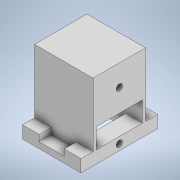
# Autodesk Inventor part: support servo
Saved by Autodesk Inventor 2022 (Build 260153000, 153)
## iProperties
Created: 2022-04-29
Part Number: support servo
Material: Generic
Document SubType Name: Modeling
Designer: Oana
Density: 1 g/cm^3
Appearance: Default
Author: Oana
Autodesk Inventor part; units mm, degrees
ref_plane "YZ Plane" through (0, 0, 0) normal (1, 0, 0) x (0, 1, 0)
ref_plane "XZ Plane" through (0, 0, 0) normal (0, 1, 0) x (-1, 0, 0)
ref_plane "XY Plane" through (0, 0, 0) normal (0, 0, 1) x (1, 0, 0)
sketch "Sketch1" plane through (0, 0, 0) normal (0, 1, 0) x (-1, 0, 0)
  line L0 (6.2884, 19.9233) -> (-5.9116, 19.9233)
  line L1 (-5.9116, 19.9233) -> (-5.9116, 12.6233)
  line L2 (-5.9116, 12.6233) -> (6.2884, 12.6233)
  line L3 (6.2884, 12.6233) -> (6.2884, 19.9233)
  point P0 (0, 0)
  dimension "d0" = 7.3
  dimension "d1" = 12.2
  constraints: 8 end point, 2 parallel, 1 horizontal, 1 perpendicular
  measures "d0" distance of L2.end L0.start
  measures "d1" distance of L0.start L0.end
extrude "Extrusion1" add sketch "Sketch1" along normal blind 3
sketch "Sketch2" plane through (0, 3, 0) normal (0, 1, 0) x (1, 0, 0)
  line L0 (5.9116, -19.9233) -> (5.9116, -12.6233) projected
  line L1 (5.9116, -12.6233) -> (-6.2884, -12.6233) projected
  line L2 (-6.2884, -12.6233) -> (-6.2884, -19.9233) projected
  line L3 (-6.2884, -19.9233) -> (5.9116, -19.9233) projected
  line L4 (5.9116, -12.6233) -> (-6.2884, -12.6233)
  line L5 (-6.2884, -12.6233) -> (-6.2884, -14.1233)
  line L6 (-6.2884, -14.1233) -> (5.9116, -14.1233)
  line L7 (5.9116, -14.1233) -> (5.9116, -12.6233)
  point P0 (0, 0)
  point P1 (5.9116, -14.1233)
  dimension "d4" = 1.5
  constraints: 8 end point, 2 parallel, 1 horizontal, 1 perpendicular, 1 point on line
  measures "d4" distance between parallel lines of L1 L6
extrude "Extrusion2" add sketch "Sketch2" along normal blind 15.7 contours L6 L2 L1 L0
sketch "Sketch3" plane through (5.9116, 0, 12.6233) normal (0, 0, -1) x (-1, 0, 0)
  line L0 (0, 0) -> (12.2, 0) projected
  line L1 (12.2, 0) -> (12.2, 18.7) projected
  line L2 (0, 18.7) -> (12.2, 18.7) projected
  line L3 (0, 0) -> (0, 18.7) projected
  line L4 (0, 18.7) -> (12.2, 18.7)
  line L5 (12.2, 18.7) -> (12.2, 15.7)
  line L6 (12.2, 15.7) -> (0, 15.7)
  line L7 (0, 15.7) -> (0, 18.7)
  point P0 (5.9116, 0)
  point P1 (0, 15.7)
  dimension "d7" = 3
  constraints: 8 end point, 2 parallel, 1 horizontal, 1 perpendicular, 1 point on line
  measures "d7" distance between parallel lines of L2 L6
extrude "Extrusion3" add sketch "Sketch3" along normal blind 23.8 contours L3 L2 L1 L6
sketch "Sketch4" plane through (-6.2884, 15.7, 12.6233) normal (0, -1, 0) x (1, 0, 0)
  line L0 (0, 0) -> (12.2, 0) projected
  line L1 (0, 0) -> (0, -23.8) projected
  line L2 (12.2, -23.8) -> (0, -23.8) projected
  line L3 (12.2, 0) -> (12.2, -23.8) projected
  line L4 (12.2, -23.8) -> (0, -23.8)
  line L5 (0, -23.8) -> (0, -22.3)
  line L6 (0, -22.3) -> (12.2, -22.3)
  line L7 (12.2, -22.3) -> (12.2, -23.8)
  point P0 (6.2884, -12.6233)
  dimension "d10" = 1.5
  constraints: 8 end point, 2 parallel, 1 horizontal, 1 perpendicular, 1 point on line
  measures "d10" distance between parallel lines of L2 L6
extrude "Extrusion4" add sketch "Sketch4" along normal up to surface (15.7 mm away) contours L6 L3 L2 L1
sketch "Sketch5" plane through (5.9116, 0, -11.1767) normal (0, 0, -1) x (-1, 0, 0)
  line L0 (12.2, 18.7) -> (12.2, 0) projected
  line L1 (12.2, 18.7) -> (0, 18.7) projected
  line L2 (0, 18.7) -> (0, 0) projected
  line L3 (12.2, 0) -> (0, 0) projected
  line L4 (12.2, 0) -> (0, 0)
  line L5 (0, 0) -> (0, 3)
  line L6 (0, 3) -> (12.2, 3)
  line L7 (12.2, 3) -> (12.2, 0)
  point P0 (5.9116, 0)
  dimension "d13" = 3
  constraints: 8 end point, 2 parallel, 1 horizontal, 1 perpendicular, 1 point on line
  measures "d13" distance between parallel lines of L3 L6
extrude "Extrusion5" add sketch "Sketch5" along normal blind 5.8 contours L0 L3 L2 L6
sketch "Sketch6" plane through (0, 0, 0) normal (0, -1, 0) x (1, 0, 0)
  arc A0 (-0.7384, -2.4741) -> (0.3616, -2.4741) centre (-0.1884, -3.4267) ccw construction
  circle A1 centre (-0.1884, -3.4267) radius 1.1 construction
  arc A2 (0.3616, -32.1794) -> (-0.7384, -32.1794) centre (-0.1884, -31.2267) ccw projected
  circle A3 centre (-0.1884, -31.2267) radius 1.5
  circle A4 centre (-0.1884, -3.4267) radius 1.5
  point P0 (0, 0)
  dimension "d16" = 3
  dimension "d17" = 3
  constraints: 3 centre point, 3 coincident, 1 concentric, 1 other
  measures "d16" diameter of A3
  measures "d17" diameter of A4
extrude "Extrusion6" cut sketch "Sketch6" against normal up to surface (3 mm away)
sketch "Sketch8" plane through (5.9116, 0, 19.9233) normal (1, 0, 0) x (0, 0, -1)
  line L0 (0, 0) -> (7.3, 0) projected
  line L1 (7.3, 0) -> (7.3, 15.7) projected
  line L2 (7.3, 15.7) -> (29.6, 15.7) projected
  line L3 (29.6, 15.7) -> (29.6, 0) projected
  line L4 (36.9, 0) -> (29.6, 0) projected
  line L5 (36.9, 3) -> (36.9, 0) projected
  line L6 (31.1, 3) -> (36.9, 3) projected
  line L7 (31.1, 18.7) -> (31.1, 3) projected
  line L8 (5.8, 18.7) -> (31.1, 18.7) projected
  line L9 (5.8, 3) -> (5.8, 18.7) projected
  line L10 (0, 3) -> (5.8, 3) projected
  line L11 (0, 0) -> (0, 3) projected
  line L12 (0, 0) -> (36.9, 0)
  line L13 (36.9, 0) -> (36.9, 6)
  line L14 (36.9, 6) -> (0, 6)
  line L15 (0, 6) -> (0, 0)
  point P0 (19.9233, 0)
  dimension "d22" = 6
  constraints: 8 end point, 2 parallel, 1 horizontal, 1 perpendicular
  measures "d22" distance of L14.end L0.start
extrude "Extrusion8" add sketch "Sketch8" along normal blind 8 contours L11 L10 L9 L14 L1 L0 | L1 L14 L3 L12 | L15 L14 L9 L10 | L3 L14 L7 L6 L5 L4 | L14 L13 L6 L7
sketch "Sketch9" plane through (-6.2884, 0, 12.6233) normal (-1, 0, 0) x (0, 0, 1)
  line L0 (-29.6, 6) -> (7.3, 6)
  line L1 (7.3, 6) -> (7.3, 0)
  line L2 (7.3, 0) -> (-29.6, 0)
  line L3 (-29.6, 0) -> (-29.6, 6)
  point P0 (-12.6233, 0)
  point P1 (7.3, 6)
  point P2 (-29.6, 0)
  constraints: 8 end point, 2 parallel, 1 horizontal, 1 perpendicular
extrude "Extrusion9" add sketch "Sketch9" along normal blind 8
sketch "Sketch10" plane through (13.9116, 0, 19.9233) normal (1, 0, 0) x (0, 0, -1)
  line L0 (0, 6) -> (0, 0) projected
  line L1 (0, 0) -> (36.9, 0) projected
  line L2 (36.9, 0) -> (36.9, 6) projected
  line L3 (36.9, 6) -> (0, 6) projected
  line L4 (0, 6) -> (36.9, 0) construction
  line L5 (36.9, 6) -> (0, 0) construction
  circle A0 centre (18.45, 3) radius 1.5
  point P0 (19.9233, 0)
  dimension "d27" = 3
  constraints: 4 end point, 1 centre point, 1 midpoint
  measures "d27" diameter of A0
extrude "Extrusion10" cut sketch "Sketch10" against normal blind 8 contours A0
sketch "Sketch11" plane through (0, 18.7, 0) normal (0, 1, 0) x (1, 0, 0)
  line L0 (5.9116, -14.1233) -> (5.9116, 11.1767) projected
  line L1 (-6.2884, 11.1767) -> (5.9116, 11.1767) projected
  line L2 (-6.2884, -14.1233) -> (-6.2884, 11.1767) projected
  line L3 (-6.2884, -14.1233) -> (5.9116, -14.1233) projected
  line L4 (5.9116, -14.1233) -> (0, -14.1233)
  line L5 (0, -14.1233) -> (0, 11.1767)
  line L6 (0, 11.1767) -> (5.9116, 11.1767)
  line L7 (5.9116, 11.1767) -> (5.9116, -14.1233)
  point P0 (0, 0)
  constraints: 8 end point, 2 parallel, 1 horizontal, 1 perpendicular, 1 point on line
extrude "Extrusion11" add sketch "Sketch11" along normal blind 10 contours L3 L5 L1 L0
sketch "Sketch12" plane through (5.9116, 15.7, 12.6233) normal (1, 0, 0) x (0, 0, -1)
  line L0 (22.3, -9.7) -> (23.8, -9.7) projected
  line L1 (23.8, -9.7) -> (23.8, 13) projected
  line L2 (-1.5, 13) -> (23.8, 13) projected
  line L3 (-1.5, -9.7) -> (-1.5, 13) projected
  line L4 (-1.5, -9.7) -> (0, -9.7) projected
  line L5 (0, -9.7) -> (0, 0) projected
  line L6 (0, 0) -> (22.3, 0) projected
  line L7 (22.3, 0) -> (22.3, -9.7) projected
  line L8 (-1.5, 13) -> (23.8, 13)
  line L9 (23.8, 13) -> (23.8, 5)
  line L10 (23.8, 5) -> (-1.5, 5)
  line L11 (-1.5, 5) -> (-1.5, 13)
  point P0 (12.6233, -15.7)
  point P1 (-1.5, 5)
  dimension "d32" = 8
  constraints: 8 end point, 2 parallel, 1 horizontal, 1 perpendicular, 1 point on line
  measures "d32" distance between parallel lines of L2 L10
extrude "Extrusion12" add sketch "Sketch12" along normal up to surface (8 mm away) contours L10 L3 L2 L1
sketch "Sketch14" plane through (0, 28.7, 0) normal (0, 1, 0) x (1, 0, 0)
  line L0 (5.9116, 11.1767) -> (5.9116, -14.1233) projected
  line L1 (0, -14.1233) -> (13.9116, -14.1233) projected
  line L2 (13.9116, -14.1233) -> (13.9116, 11.1767) projected
  line L3 (0, 11.1767) -> (13.9116, 11.1767) projected
  line L4 (0, 11.1767) -> (0, -14.1233) projected
  line L5 (0, 11.1767) -> (13.9116, 11.1767)
  line L6 (13.9116, 11.1767) -> (13.9116, -14.1233)
  line L7 (13.9116, -14.1233) -> (0, -14.1233)
  line L8 (0, -14.1233) -> (0, 11.1767)
  point P0 (0, 0)
  constraints: 8 end point, 2 parallel, 1 horizontal, 1 perpendicular
extrude "Extrusion14" add sketch "Sketch14" along normal blind 8
sketch "Sketch16" plane through (5.9116, 15.7, 12.6233) normal (1, 0, 0) x (0, 0, -1)
  line L0 (23.8, 5) -> (-1.5, 5) projected
  line L1 (-1.5, -9.7) -> (-1.5, 5) projected
  line L2 (-1.5, -9.7) -> (0, -9.7) projected
  line L3 (0, -9.7) -> (0, 0) projected
  line L4 (0, 0) -> (22.3, 0) projected
  line L5 (22.3, 0) -> (22.3, -9.7) projected
  line L6 (22.3, -9.7) -> (23.8, -9.7) projected
  line L7 (23.8, -9.7) -> (23.8, 5) projected
  point P0 (12.6233, -15.7)
extrude "Extrusion16" add sketch "Sketch16" along normal blind 8
sketch "Sketch17" plane through (13.9116, 0, 19.9233) normal (1, 0, 0) x (0, 0, -1)
  circle A0 centre (18.45, 3) radius 1.5 projected
  line L0 (18.45, 3) -> (18.45, 26.5)
  circle A1 centre (18.45, 26.5) radius 1.5
  point P0 (19.9233, 0)
  dimension "d46" = 23.5
  dimension "d47" = 3
  constraints: 2 end point, 1 centre point, 1 coincident, 1 vertical
  measures "d46" distance of L0.start L0.end
  measures "d47" diameter of A1
extrude "Extrusion17" cut sketch "Sketch17" against normal blind 8 contours A1
sketch "Sketch18" plane through (0, 18.7, -11.1767) normal (-1, 0, 0) x (0, 0, 1)
  line L0 (25.3, 0) -> (0, 0) projected
  line L1 (25.3, 0) -> (25.3, 18) projected
  line L2 (0, 18) -> (25.3, 18) projected
  line L3 (0, 0) -> (0, 18) projected
  line L4 (0, -12.7) -> (1.5, -12.7) projected
  line L5 (1.5, -3) -> (1.5, -12.7) projected
  line L6 (23.8, -3) -> (1.5, -3) projected
  line L7 (23.8, -12.7) -> (23.8, -3) projected
  line L8 (23.8, -12.7) -> (25.3, -12.7) projected
  line L9 (25.3, -12.7) -> (25.3, 0) projected
  line L10 (25.3, 0) -> (0, 0) projected
  line L11 (0, 0) -> (0, -12.7) projected
  point P0 (11.1767, -18.7)
extrude "Extrusion18" add sketch "Sketch18" along normal up to surface (14.2884 mm away) contours L0 L3 L2 L1
sketch "Sketch19" plane through (-6.2884, 15.7, -9.6767) normal (-1, 0, 0) x (0, 0, 1)
  line L0 (-1.5, -9.7) -> (0, -9.7) projected
  line L1 (0, 0) -> (0, -9.7) projected
  line L2 (22.3, 0) -> (0, 0) projected
  line L3 (22.3, -9.7) -> (22.3, 0) projected
  line L4 (22.3, -9.7) -> (23.8, -9.7) projected
  line L5 (23.8, -9.7) -> (23.8, 3) projected
  line L6 (23.8, 3) -> (-1.5, 3) projected
  line L7 (-1.5, 3) -> (-1.5, -9.7) projected
  point P0 (9.6767, -15.7)
extrude "Extrusion19" add sketch "Sketch19" along normal up to surface (8 mm away)
sketch "Sketch20" plane through (-14.2884, 0, 12.6233) normal (-1, 0, 0) x (0, 0, 1)
  line L0 (-23.8, 6) -> (-29.6, 6) projected
  line L1 (-29.6, 6) -> (-29.6, 0) projected
  line L2 (-29.6, 0) -> (7.3, 0) projected
  line L3 (7.3, 0) -> (7.3, 6) projected
  line L4 (7.3, 6) -> (1.5, 6) projected
  line L5 (1.5, 36.7) -> (1.5, 6) projected
  line L6 (-23.8, 36.7) -> (1.5, 36.7) projected
  line L7 (-23.8, 6) -> (-23.8, 36.7) projected
  line L8 (-22.3, 15.7) -> (-22.3, 6) projected
  line L9 (0, 15.7) -> (-22.3, 15.7) projected
  line L10 (0, 6) -> (0, 15.7) projected
  line L11 (0, 6) -> (-22.3, 6) projected
  line L12 (-29.6, 6) -> (7.3, 0) construction
  line L13 (7.3, 6) -> (-29.6, 0) construction
  circle A0 centre (-11.15, 3) radius 1.5
  point P0 (-12.6233, 0)
  dimension "d54" = 3
  constraints: 4 end point, 1 centre point, 1 midpoint
  measures "d54" diameter of A0
extrude "Extrusion20" cut sketch "Sketch20" against normal blind 8 contours A0
sketch "Sketch21" plane through (-14.2884, 0, 12.6233) normal (-1, 0, 0) x (0, 0, 1)
  circle A0 centre (-11.15, 26.5) radius 1.5 projected
  point P0 (-12.6233, 0)
extrude "Extrusion21" cut sketch "Sketch21" against normal blind 8
body "Solid1"
